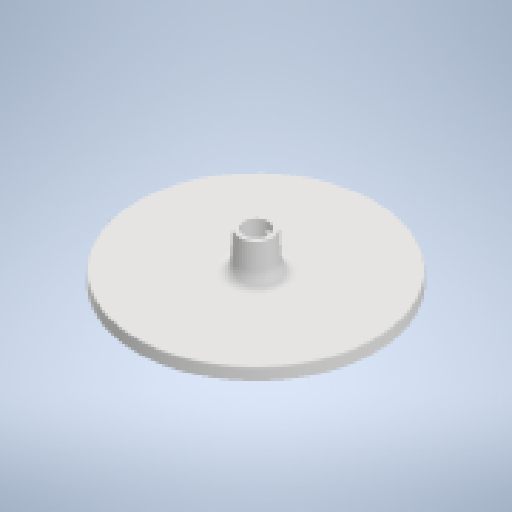
# Autodesk Inventor part: Pie2
Saved by Autodesk Inventor 2024 (Build 280153000, 153)
## iProperties
Created: 2023-12-01
Part Number: Pie2
Material: Genérico
Document SubType Name: Modeling
Designer: sergi
Density: 1 g/cm^3
Appearance: Valor por defecto
Author: sergi
Autodesk Inventor part; units mm, degrees
ref_plane "YZ Plane" through (0, 0, 0) normal (1, 0, 0) x (0, 1, 0)
ref_plane "XZ Plane" through (0, 0, 0) normal (0, 1, 0) x (-1, 0, 0)
ref_plane "XY Plane" through (0, 0, 0) normal (0, 0, 1) x (1, 0, 0)
sketch "Boceto2" plane through (0, 0, 0) normal (0, 1, 0) x (-1, 0, 0)
  circle A0 centre (0, 0) radius 100
  dimension "d11" = 200
  constraints: 1 centre point, 1 coincident
  measures "d11" diameter of A0
extrude "Extrusión2" add sketch "Boceto2" along normal blind 10
sketch "Boceto3" plane through (0, 10, 0) normal (0, 1, 0) x (1, 0, 0)
  circle A0 centre (0, 0) radius 100 projected
  constraints: 1 coincident
hole "Agujero1" at (0, 10, 0) direction (0, -1, 0) diameter 20.5 depth 7
sketch "Boceto4" plane through (0, 10, 0) normal (0, 1, 0) x (1, 0, 0)
  circle A0 centre (0, 0) radius 10.25 projected
  circle A1 centre (0, 0) radius 100 projected
  circle A2 centre (0, 0) radius 15.25
  dimension "d21" = 5
  constraints: 1 centre point
  measures "d21" radial gap between concentric circles of A0 A2
extrude "Extrusión3" add sketch "Boceto4" along normal blind 30 contours A2
sketch "Boceto5" plane through (0, 0, 0) normal (0, 0, 1) x (1, 0, 0)
  line L0 (15.25, 40) -> (-15.25, 40) projected
  line L1 (0, 40) -> (0, 20)
  line L2 (0, 40) -> (0, 31.6087)
  line L3 (0, 31.6087) -> (0, 23.2173)
  circle A0 centre (0, 23.2173) radius 2.25
  circle A1 centre (0, 31.6087) radius 2.25
  point P0 (0, 0)
  point P1 (-15.25, 20)
  point P2 (15.25, 20)
  dimension "d25" = 8.3913
  dimension "d26" = 8.3913
  dimension "d27" = 4.5
  dimension "d28" = 4.5
  constraints: 6 end point, 2 centre point, 2 coincident, 2 point on line, 1 midpoint
  measures "d25" distance of L1.start L2.end
  measures "d26" distance of L2.end L3.end
  measures "d27" diameter of A0
  measures "d28" diameter of A1
fillet "Empalme2" radius 1 1 edges at (100, 10, 0)
chamfer "Chaflán1" distance 30 angle 3 1 edges at (-15.25, 40, 0) measured on face at (15.2005, 30, 1.2271)
hole "Agujero3" at (0, 31.6087, 0) at (0, 23.2173, 0) direction (0, 0, -1) diameter 4.5 end through all
fillet "Empalme3" radius 10 2 edges at (-15.25, 10.0005, 0) (-15.25, 10, 0)
sketch "Boceto6" plane through (0, 0, 0) normal (0, -1, 0) x (1, 0, 0)
  circle A0 centre (0, 0) radius 100 projected
  circle A1 centre (0, 0) radius 5
  line L0 (5, 0) -> (5, -105)
  line L1 (-5, 0) -> (-5, -105)
  point P0 (-5, -99.8749)
  point P1 (5, -99.8749)
  dimension "d48" = 10
  dimension "d49" = 105
  dimension "d50" = 10
  constraints: 4 end point, 1 coincident, 1 parallel, 1 vertical, 3 other
  measures "d49" distance of L0.start L0.end
  measures "d50" distance between parallel lines of L0 L1
extrude "Extrusión4" cut sketch "Boceto6" against normal blind 5 contours L1 A1 L0 A0 | A1 picked at (0.2009, -68.3119)
sketch "Boceto7" plane through (-5, 0, 0) normal (1, 0, 0) x (0, 0, -1)
  point P0 (0, 0)
fillet "Empalme4" radius 2 2 edges at (-5, 5, -54.4113) (5, 5, -54.4113)
